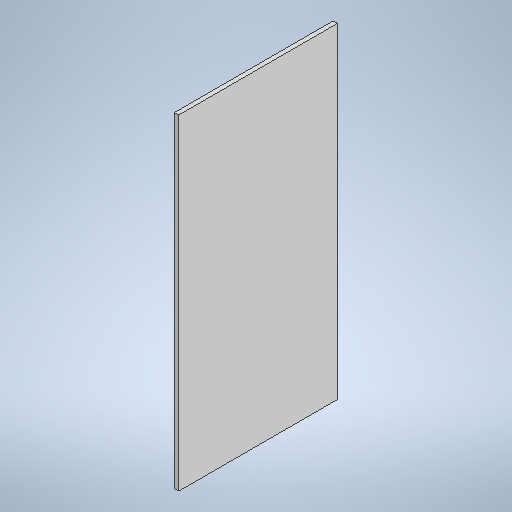
# Autodesk Inventor part: 가로로만 옆판
Saved by Autodesk Inventor 2025.1 (Build 291241000, 241)
## iProperties
Created: 2024-10-29
Part Number: 가로로만 옆판
Material: 일반
Document SubType Name: Modeling
Designer: gmsee
Density: 1 g/cm^3
Appearance: 기본값
Author: gmsee
Autodesk Inventor part; units mm, degrees
ref_plane "YZ Plane" through (0, 0, 0) normal (1, 0, 0) x (0, 1, 0)
ref_plane "XZ Plane" through (0, 0, 0) normal (0, 1, 0) x (-1, 0, 0)
ref_plane "XY Plane" through (0, 0, 0) normal (0, 0, 1) x (1, 0, 0)
sketch "스케치1" plane through (0, 0, 0) normal (1, 0, 0) x (0, 1, 0)
  line L0 (76, 37) -> (-76, 37)
  line L1 (-76, 37) -> (-76, -37)
  line L2 (-76, -37) -> (76, -37)
  line L3 (76, -37) -> (76, 37)
  point P0 (0, 0)
  dimension "d0" = 152
  dimension "d1" = 74
  dimension "d2" = 37
  dimension "d3" = 76
  constraints: 8 end point, 2 parallel, 1 horizontal, 1 perpendicular
  measures "d0" distance between parallel lines of L1 L3
  measures "d1" distance between parallel lines of L2 L0
  measures "d2" distance from line of L2 point (0, 0)
  measures "d3" distance from line of L1 point (0, 0)
extrude "돌출1" add sketch "스케치1" along normal blind 2
equation "\"d2\" = 0.5 * d1"
equation "\"d3\" = 0.5 * d0"
